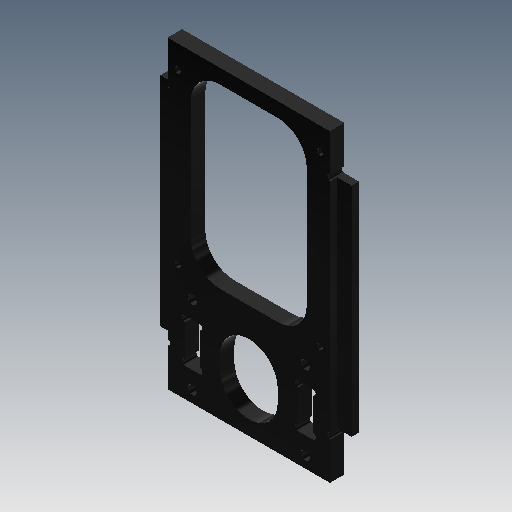
# Autodesk Inventor part: コックピット_2_サブフレーム_1
Saved by Autodesk Inventor 2017.3 (Build 213256000, 256)
## iProperties
Created: 2016-05-24
Part Number: コックピット_2_サブフレーム_1
Material: アセタール樹脂、黒
Document SubType Name: Modeling
Designer: hiroaki
Density: 1.425 g/cm^3
Appearance: 滑らか - 黒
Mass: 23.4277 g
Surface Area: 110.659 cm^2
Volume: 16.4405 cm^3
Author: hiroaki
Autodesk Inventor part; units mm, degrees
ref_plane "YZ Plane" through (0, 0, 0) normal (1, 0, 0) x (0, 1, 0)
ref_plane "XZ Plane" through (0, 0, 0) normal (0, 1, 0) x (-1, 0, 0)
ref_plane "XY Plane" through (0, 0, 0) normal (0, 0, 1) x (1, 0, 0)
sketch "スケッチ1" plane through (0, 0, 0) normal (0, 0, 1) x (1, 0, 0)
  line L0 (-28, -52.5) -> (28, -52.5) construction
  line L1 (28, -52.5) -> (28, 52.5) construction
  line L2 (28, 52.5) -> (-28, 52.5) construction
  line L3 (-28, 52.5) -> (-28, -52.5) construction
  line L4 (-28, -52.5) -> (28, 52.5) construction
  line L5 (28, -52.5) -> (-28, 52.5) construction
  line L6 (-28, 39.6) -> (-28, 52.5)
  line L7 (-28, 52.5) -> (28, 52.5)
  line L8 (28, 52.5) -> (28, 39.6)
  line L9 (-28, 37.5) -> (-33, 37.5)
  line L10 (-33, 37.5) -> (-33, -37.5)
  line L11 (-33, -37.5) -> (-28, -37.5)
  line L12 (-28, -39.6) -> (-28, -52.5)
  line L13 (-28, -52.5) -> (28, -52.5)
  line L14 (28, -52.5) -> (28, -39.6)
  line L15 (28, 37.5) -> (33, 37.5)
  line L16 (33, 37.5) -> (33, -37.5)
  line L17 (33, -37.5) -> (28, -37.5)
  arc A0 (-28, 37.5) -> (-28, 39.6) centre (-28, 38.55) ccw
  arc A1 (-28, -39.6) -> (-28, -37.5) centre (-28, -38.55) ccw
  arc A2 (28, -37.5) -> (28, -39.6) centre (28, -38.55) ccw
  line L18 (0, 0) -> (0, 52.5) construction
  line L19 (0, 0) -> (28, 0) construction
  arc A3 (28, 39.6) -> (28, 37.5) centre (28, 38.55) ccw
  line L20 (-24.5, 44.5) -> (24.5, 44.5) construction
  line L21 (24.5, 44.5) -> (24.5, -13.5) construction
  line L22 (24.5, -13.5) -> (-24.5, -13.5) construction
  line L23 (-24.5, -13.5) -> (-24.5, 44.5) construction
  line L24 (-24.5, 44.5) -> (24.5, -13.5) construction
  line L25 (24.5, 44.5) -> (-24.5, -13.5) construction
  circle A4 centre (-24.5, 44.5) radius 1.04
  circle A5 centre (-24.5, -13.5) radius 1.04
  circle A6 centre (24.5, -13.5) radius 1.04
  circle A7 centre (24.5, 44.5) radius 1.04
  line L26 (-22, -27.5) -> (-17, -27.5) construction
  line L27 (-17, -27.5) -> (-17, -42.5) construction
  line L28 (-17, -42.5) -> (-22, -42.5) construction
  line L29 (-22, -42.5) -> (-22, -27.5) construction
  circle A8 centre (-19.5, -21.5) radius 1.55
  circle A9 centre (-19.5, -48.5) radius 1.55
  line L30 (-17, -35) -> (-22, -35) construction
  line L31 (-22, -17.5) -> (-17, -17.5) construction
  line L32 (-17, -17.5) -> (-17, -52.5) construction
  line L33 (-17, -52.5) -> (-22, -52.5) construction
  line L34 (-22, -52.5) -> (-22, -17.5) construction
  circle A10 centre (-19.5, -48.5) radius 3 construction
  line L35 (-16.95, -27.45) -> (-22.05, -27.45)
  line L36 (-22.05, -27.45) -> (-22.05, -42.55)
  line L37 (-22.05, -42.55) -> (-16.95, -42.55)
  line L38 (-16.95, -42.55) -> (-16.95, -27.45)
  circle A11 centre (-22.05, -28.5) radius 1.05
  circle A12 centre (-16.95, -28.5) radius 1.05
  circle A13 centre (-22.05, -41.5) radius 1.05
  circle A14 centre (-16.95, -41.5) radius 1.05
  circle A15 centre (19.5, -21.5) radius 1.55
  circle A16 centre (19.5, -48.5) radius 1.55
  line L39 (16.95, -27.45) -> (22.05, -27.45)
  line L40 (22.05, -27.45) -> (22.05, -42.55)
  line L41 (22.05, -42.55) -> (16.95, -42.55)
  line L42 (16.95, -42.55) -> (16.95, -27.45)
  circle A17 centre (22.05, -28.5) radius 1.05
  circle A18 centre (16.95, -28.5) radius 1.05
  circle A19 centre (22.05, -41.5) radius 1.05
  circle A20 centre (16.95, -41.5) radius 1.05
  point P0 (0, 15.5)
  point P1 (0, 15.5)
  point P2 (0, 0)
  point P3 (-19.5, -35)
  point P4 (-19.5, -17.5)
  dimension "d93" = 2.1
  dimension "d9" = 56
  dimension "d12" = 105
  dimension "d13" = 15
  dimension "d39" = 15
  dimension "d40" = 1.05
  dimension "d41" = 5
  dimension "d52" = 2.08
  dimension "d53" = 49
  dimension "d54" = 58
  dimension "d55" = 8
  dimension "d73" = 35
  dimension "d83" = 5
  dimension "d87" = 3.1
  dimension "d88" = 10
  dimension "d89" = 27
  dimension "d90" = 6
  dimension "d91" = 22
  dimension "d92" = 0.05
  constraints: 86 end point, 16 symmetric about line, 14 perpendicular, 13 centre point, 13 midpoint, 12 point on line, 12 vertical alignment, 10 parallel, 8 point on circle, 6 collinear, 6 horizontal, 6 vertical, 5 coincident, 5 equal radius, 3 horizontal alignment, 1 tangent, 22 other
  measures "d9" distance of L1.end L2.end
  measures "d12" distance of L0.end L1.end
  measures "d13" distance between parallel lines of L9 L2
  measures "d39" distance between parallel lines of L0 L11
  measures "d40" radius of A0
  measures "d41" distance of L9.start L9.end
  measures "d52" diameter of A4
  measures "d53" distance of L20.start L20.end
  measures "d54" distance of L22.end L20.start
  measures "d55" distance between parallel lines of L2 L20
  measures "d73" distance of L31.end L32.end
  measures "d83" distance of L31.start L31.end
  measures "d87" diameter of A8
  measures "d88" distance between parallel lines of L31 L26
  measures "d89" distance of A9.centre A8.centre
  measures "d90" diameter of A10
  measures "d91" distance between parallel lines of L18 L34
  measures "d92" distance between parallel lines of L35 L26
extrude "押し出し1" add sketch "スケッチ1" along normal blind 5
sketch "スケッチ2" plane through (0, 0, 5) normal (0, 0, 1) x (1, 0, 0)
  line L0 (-28, 52.5) -> (-28, 39.6) projected
  line L1 (28, 52.5) -> (-28, 52.5) projected
  line L2 (-67.7785, 43.014) -> (-28, 43.014)
  line L3 (-28, 43.014) -> (-28, -43.014)
  line L4 (-28, -43.014) -> (-67.7785, -43.014)
  line L5 (-67.7785, -43.014) -> (-67.7785, 43.014)
  line L6 (67.7785, 43.014) -> (28, 43.014)
  line L7 (28, 43.014) -> (28, -43.014)
  line L8 (28, -43.014) -> (67.7785, -43.014)
  line L9 (67.7785, -43.014) -> (67.7785, 43.014)
  line L10 (0, 0) -> (0, 52.5) construction
  line L11 (0, 0) -> (33, 0) construction
  line L12 (33, 37.5) -> (33, -37.5) construction
  constraints: 20 end point, 4 parallel, 2 horizontal, 2 midpoint, 2 perpendicular, 2 symmetric about line, 1 collinear, 3 other
extrude "押し出し2" cut sketch "スケッチ2" against normal blind 2.5
sketch "スケッチ4" plane through (0, 0, 5) normal (0, 0, 1) x (1, 0, 0)
  line L0 (28, 52.5) -> (-28, 52.5) projected
  line L1 (-28, 52.5) -> (-28, 39.6) projected
  line L2 (-28, -52.5) -> (28, -52.5) projected
  line L3 (-16.95, -42.55) -> (-22.05, -42.55) projected
  arc A0 (-22.05, -40.45) -> (-22.05, -42.55) centre (-22.05, -41.5) ccw projected
  line L4 (-22.05, -40.45) -> (-22.05, -29.55) projected
  arc A1 (-22.05, -27.45) -> (-22.05, -29.55) centre (-22.05, -28.5) ccw projected
  line L5 (-22.05, -27.45) -> (-16.95, -27.45) projected
  arc A2 (-16.95, -29.55) -> (-16.95, -27.45) centre (-16.95, -28.5) ccw projected
  line L6 (-16.95, -29.55) -> (-16.95, -40.45) projected
  arc A3 (-16.95, -42.55) -> (-16.95, -40.45) centre (-16.95, -41.5) ccw projected
  circle A4 centre (-19.5, -21.5) radius 1.55 projected
  line L7 (-20, 47.5) -> (20, 47.5)
  line L8 (20, 47.5) -> (20, -13.5)
  line L9 (20, -13.5) -> (-20, -13.5)
  line L10 (-20, -13.5) -> (-20, 47.5)
  line L11 (-10, -23.5) -> (10, -23.5)
  line L12 (10, -23.5) -> (10, -47.5)
  line L13 (10, -47.5) -> (-10, -47.5)
  line L14 (-10, -47.5) -> (-10, -23.5)
  line L15 (-16.95, -27.5) -> (-22.05, -27.5) construction
  arc A5 (-22.05, -27.5) -> (-22, -29.4987) centre (-22.05, -28.5) ccw construction
  line L16 (-22, -29.4987) -> (-22, -40.5013) construction
  arc A6 (-22, -40.5013) -> (-22.05, -42.5) centre (-22.05, -41.5) ccw construction
  line L17 (-22.05, -42.5) -> (-16.95, -42.5) construction
  arc A7 (-16.95, -42.5) -> (-17, -40.5013) centre (-16.95, -41.5) ccw construction
  line L18 (-17, -40.5013) -> (-17, -29.4987) construction
  arc A8 (-17, -29.4987) -> (-16.95, -27.5) centre (-16.95, -28.5) ccw construction
  point P0 (0, 0)
  point P1 (0, 47.5)
  point P2 (0, -13.5)
  point P3 (0, -23.5)
  dimension "d94" = 8
  dimension "d95" = 5
  dimension "d96" = 8
  dimension "d97" = 0.05
  dimension "d98" = 7
  dimension "d99" = 5
  dimension "d100" = 10
  constraints: 24 end point, 8 point on circle, 4 centre point, 4 parallel, 3 midpoint, 2 horizontal, 2 perpendicular, 2 vertical alignment, 7 other
  measures "d94" distance between parallel lines of L1 L10
  measures "d95" distance between parallel lines of L0 L7
  measures "d96" distance from line of A4.centre L9
  measures "d97" distance between parallel lines of L6 L18
  measures "d98" distance between parallel lines of L14 L18
  measures "d99" distance between parallel lines of L2 L13
  measures "d100" distance between parallel lines of L9 L11
extrude "押し出し4" cut sketch "スケッチ4" against normal blind 10 contours L7 L8 L9 L10 | L11 L12 L13 L14
fillet "フィレット2" radius 10 8 edges at (-10, -47.5, 2.5) (-10, -23.5, 2.5) (10, -23.5, 2.5) (10, -47.5, 2.5) (-20, -13.5, 2.5) (-20, 47.5, 2.5) (20, 47.5, 2.5) (20, -13.5, 2.5)
equation "\"d12\" = d19"
equation "\"d13\" = d26"
equation "\"d39\" = d27"
equation "\"d55\" = d69"
equation "\"d73\" = d1_1_2 + 2 * d2_1"
equation "\"d88\" = d2_1"
equation "\"d99\" = d95"
equation "\"d19\" = 105"
equation "\"d26\" = 15"
equation "\"d27\" = 15"
equation "\"d69\" = 8"
equation "\"d1_1_2\" = 15"
equation "\"d2_1\" = 10"
